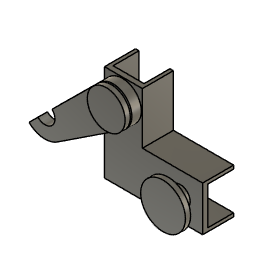
CornerLatch (Autodesk Fusion 360 design; units mm, degrees)
Autodesk Fusion 360 part; units mm, degrees
sketch "Sketch1" plane through (0, 0, 0) normal (0, 0, 1) x (1, 0, 0)
  line L0 (0, 0) -> (57, 0)
  line L1 (57, 0) -> (57, 26)
  line L2 (57, 26) -> (22, 26)
  line L3 (22, 26) -> (22, 56)
  line L4 (0, 56) -> (0, 0)
  line L5 (57, 26) -> (22, 26)
  line L6 (57, 24) -> (57, 26)
  line L7 (57, 0) -> (29.1762, 0)
  line L8 (57, 2) -> (57, 0)
  line L9 (22, 56) -> (22, 26)
  circle A0 centre (11, 45) radius 6.0047
  circle A1 centre (11, 45) radius 6.8331
  circle A2 centre (11, 45) radius 11
  circle A3 centre (44, 13) radius 5.7803
  circle A4 centre (44, 13) radius 13
  line L10 (18.3068, 53.2226) -> (52.6353, 22.7176)
  line L11 (20, 2) -> (20, 0)
  line L12 (20, 2) -> (57, 2)
  line L13 (20, 24) -> (57, 24)
  line L14 (20, 24) -> (20, 56)
  line L15 (2, 0) -> (2, 56)
  line L16 (0, 56) -> (22, 56)
  line L17 (44, 13) -> (5.4546, 35.5001)
  line L18 (44, 13) -> (55.2272, 6.4464)
  dimension "d28" = 2
  dimension "d29" = 2
  dimension "d50" = 18
  dimension "d51" = 2
  dimension "d52" = 2
  dimension "d54" = 22
  dimension "d55" = 18
  dimension "d57" = 35
  dimension "d58" = 30
  constraint coincident L0.start L4.end
  constraint horizontal L0
  constraint perpendicular L0 L1
  constraint perpendicular L1 L2
  constraint perpendicular L2 L3
  constraint perpendicular L0 L4
  constraint horizontal L5
  constraint vertical L6
  constraint horizontal L7
  constraint vertical L8
  constraint coincident A4 L10.end
  constraint coincident L0 L11.end
  constraint perpendicular L0 L11
  constraint perpendicular L1 L13
  constraint parallel L12 L13
  constraint coincident L0 L15.start
  constraint tangent L3 A2
  constraint concentric A1 A2
  constraint concentric A0 A1
  constraint perpendicular L3 L16
  constraint coincident L16 L15.end
  constraint coincident L16 L14.end
  constraint tangent A2 L16
  constraint coincident A2 L10.start
  constraint tangent A2 L10
  constraint tangent L4 A2
  constraint tangent A4 L10
  constraint tangent L0 A4
  constraint tangent L5 A4
  constraint tangent L1 A4
  constraint concentric A3 A4
  constraint coincident A3.centre A4.centre
  constraint coincident A2 L17.end
  constraint tangent A2 L17
  constraint coincident A4 L18.end
  constraint parallel L17 L18
  measures "d28" distance of L11.start L11.end
  measures "d29" distance of L2 L13
  measures "d50" distance of L11 L15
  measures "d51" distance of L4 L15
  measures "d52" distance of L9 L14
  measures "d54" distance of L12 L13
  measures "d55" distance of L14 L15
  measures "d57" distance of L1.end L2.end
  measures "d58" distance of L2.end L3.end
extrude "Extrude1" add sketch "Sketch1" along normal blind 3 contours L0 L4 A2 L15 | L0 A2 A4 L11 L12 L13 L14 L15 L17 | L4 A2 L15 L16 | A2 L15 | L0 L7 A4 L11 L12 | A2 L14 L15 | A2 L15 L16 | A2 L14 L17 | A2 L10 L14 L16 | L0 L1 L7 L8 A4 L12 | A4 L12 | A3 A4 L12 L17 L18 | A2 L14 | L2 L3 L5 L9 A2 A4 L13 L14 L17 | L13 L14 L17 | A2 L10 L14 | L3 L9 L10 L14 L16 | L1 A4 L12 | A4 L13 L17 | A3 A4 L13 L17 L18 | L3 L9 A2 L10 L14 | A4 L13 | A3 L17 L18 | A3 L17 L18 | L1 A4 L10 L13 | L2 L5 A4 L10 L13 | A4 L10 L13 | L1 L2 L5 L6 L10 L13 | A0 | A1 makes body 1
extrude "Extrude2" add sketch "Sketch1" against normal blind 15 contours L0 L4 A2 L15 | L4 A2 L15 L16 | A2 L15 | L0 L7 A4 L11 L12 | L0 L1 L7 L8 A4 L12 | A4 L12 | A2 L14 | L2 L3 L5 L9 A2 A4 L13 L14 L17 | L13 L14 L17 | L3 L9 L10 L14 L16 | L3 L9 A2 L10 L14 | A4 L13 | L2 L5 A4 L10 L13 | L1 L2 L5 L6 L10 L13 bodies 1
extrude "Extrude3" add sketch "Sketch1" along normal blind 10 contours A3 L17 L18 | A3 L17 L18 | A0 bodies 1
extrude "Extrude4" add sketch "Sketch1" along normal blind 3 from surface at 10 contours A2 L15 | A2 L14 L15 | A4 L12 | A3 A4 L12 L17 L18 | A2 L14 | A3 A4 L13 L17 L18 | A4 L13 | A3 L17 L18 | A3 L17 L18 | A0 | A1 bodies 1
extrude "Extrude5" add sketch "Sketch1" along normal blind 5.5 from surface at 3.6 separate body contours A2 L15 | A2 L14 L15 | A2 L14 L17 | A2 L14 | L2 L3 L5 L9 A2 A4 L13 L14 L17 | A2 L10 L14 | A4 L13 L17 | A3 A4 L13 L17 L18 | L2 L3 L5 L9 L10 | L3 L9 A2 L10 L14 | A4 L13 | L2 L5 A4 L10 L13 | A4 L10 L13 makes body 2
move_body "Move1" bodies 2 to x (-0.258819, -0.965926, 0) y (0.965926, -0.258819, 0) z (0, 0, 1) at (-29.6197, 67.272, 0)
move_body "Move2" bodies 2 1 to x (1, 0, 0) y (0, 0, 1) z (0, -1, 0) at (0, 3, 3)
move_body "Move4" bodies 2 1 to x (1, 0, 0) y (0, 1, 0) z (0, 0, 1) at (0, 0, -3)
sketch "Sketch8" plane through (0, -0.6, 0) normal (0, 1, 0) x (-1, 0, 0)
  circle A0 centre (-11, 45) radius 6.8331
  line L0 (37.6868, 12.2582) -> (32.5574, 17.3389)
  arc A1 (24.3439, 25.4744) -> (32.5574, 17.3389) centre (28.4507, 21.4067) ccw
  line L1 (24.3439, 25.4744) -> (-3.259, 52.8152)
  arc A2 (-3.259, 52.8152) -> (-17.0513, 35.814) centre (-11, 45) ccw
  line L2 (-17.0513, 35.814) -> (21.2991, 10.5505)
  arc A3 (21.2991, 10.5505) -> (37.6868, 12.2582) centre (28.4507, 21.4067) ccw
  line L3 (10.5425, 39.1448) -> (2.1239, 23.1823)
  circle A4 centre (6.3332, 31.1635) radius 5
  dimension "d62" = 10
  constraint midpoint L1 L3.start
  constraint midpoint L2 L3.end
  constraint midpoint L3 A4.centre
  measures "d62" diameter of A4
extrude "Extrude11" add sketch "Sketch8" along normal blind 4 contours L3 A4 | L3 A4 bodies 2
